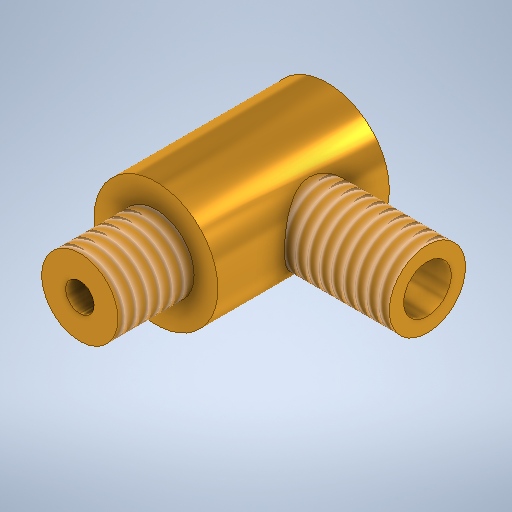
# Autodesk Inventor part: 157
Saved by Autodesk Inventor 2025.1 (Build 291241000, 241)
## iProperties
Created: 2024-08-03
Part Number: 157
Material: Iron, Cast
Document SubType Name: Modeling
Designer: ffogue
Density: 7.15 g/cm^3
Appearance: Metal 1800F Hot
Author: ffogue
Autodesk Inventor part; units mm, degrees
ref_plane "XZ Plane" through (0, 0, 0) normal (0, 1, 0) x (-1, 0, 0)
ref_plane "XY Plane" through (0, 0, 0) normal (0, 0, 1) x (1, 0, 0)
sketch "Sketch1" plane through (0, 0, 0) normal (0, 0, 1) x (1, 0, 0)
  line L0 (0, 0) -> (0, 26)
  line L1 (0, 26) -> (6.5, 26)
  line L2 (6.5, 26) -> (6.5, 8)
  line L3 (6.5, 8) -> (4, 8)
  line L4 (4, 8) -> (4, 0)
  line L5 (4, 0) -> (0, 0)
  dimension "d0" = 13
  dimension "d1" = 8
  dimension "d2" = 8
  dimension "d3" = 18
  constraints: 12 end point, 5 perpendicular, 1 vertical
  measures "d0" diameter of L2 L0
  measures "d1" diameter of L4 L0
  measures "d2" distance of L3.end L4.end
  measures "d3" distance of L1.end L2.end
revolve "Revolution1" add sketch "Sketch1" angle 360 about axis through (0, 0, 0) along (0, 1, 0)
thread "Thread1" size "M8x1.25" class "6g" standard "ISO Metric profile" full length
ref_plane "Work Plane1" through (17.5, 0, 0) normal (1, 0, 0) x (0, 1, 0)
sketch "Sketch2" plane through (17.5, 0, 0) normal (1, 0, 0) x (0, 1, 0)
  line L0 (26, -6.5) -> (26, 6.5) projected
  line L1 (8, 6.5) -> (26, 6.5) projected
  line L2 (8, -6.5) -> (26, -6.5) projected
  line L3 (8, -6.5) -> (8, 6.5) projected
  circle A0 centre (19, 0) radius 4
  point P0 (0, 0)
  point P1 (26, 0)
  dimension "d8" = 8
  dimension "d9" = 7
  constraints: 1 centre point, 1 horizontal alignment, 1 midpoint
  measures "d8" diameter of A0
  measures "d9" distance from line of L0 A0.centre
extrude "Extrusion1" add sketch "Sketch2" against normal up to surface contours A0
sketch "Sketch3" plane through (17.5, 19, 0) normal (1, 0, 0) x (0, 0, -1)
  circle A0 centre (0, 0) radius 4 projected
  point P0 (0, -19)
  constraints: 1 coincident
hole "Hole1" at (17.5, 19, 0) direction (-1, 0, 0) diameter 4 depth 17.5 counterbore diameter 5 counterbore depth 10
sketch "Sketch4" plane through (0, 0, 0) normal (0, -1, 0) x (1, 0, 0)
  circle A0 centre (0, 0) radius 4 projected
  point P0 (0, 0)
  constraints: 1 coincident
hole "Hole2" at (0, 0, 0) direction (0, 1, 0) diameter 3 depth 20
thread "Thread2" size "M8x1.25" class "6g" standard "ISO Metric profile" length 15
body "Solid1"
